Corner Structure (Autodesk Fusion 360 design; units mm, degrees)
Autodesk Fusion 360 part; units mm, degrees
sketch "Sketch1" plane through (0, 0, 0) normal (0, 0, 1) x (1, 0, 0)
  line L0 (0, 0) -> (-45, 0)
  line L1 (0, 0) -> (0, 45)
  line L2 (0, 45) -> (-45, 0)
  line L3 (-5, 40) -> (-5, 5)
  line L4 (-5, 5) -> (-40, 5)
  line L5 (-2, 43) -> (0, 43)
  line L6 (-43, 2) -> (-43, 0)
  dimension "d1" = 45
  dimension "d2" = 45
  dimension "d5" = 5
  dimension "d6" = 5
  dimension "d7" = 2
  dimension "d8" = 2
  constraint coincident L0.start L1.start
  constraint horizontal L0
  constraint perpendicular L0 L1
  constraint coincident L2 L3.start
  constraint parallel L1 L3
  constraint coincident L2 L4.end
  constraint perpendicular L3 L4
  constraint coincident L2 L5.start
  constraint coincident L1 L5.end
  constraint perpendicular L1 L5
  constraint coincident L2 L6.start
  constraint coincident L0 L6.end
  constraint perpendicular L0 L6
  measures "d1" distance of L0.start L0.end
  measures "d2" distance of L0.start L1.end
  measures "d5" vertical distance of L0.start L3.end
  measures "d6" horizontal distance of L0.start L3.end
  measures "d7" distance of L0.end L6.end
  measures "d8" distance of L1.end L5.end
extrude "Extrude2" add sketch "Sketch1" along normal blind 20 contours L0 L1 L2 L3 L4 L5 L6
extrude "Extrude3" add sketch "Sketch1" along normal blind 5 contours L2 L3 L4
